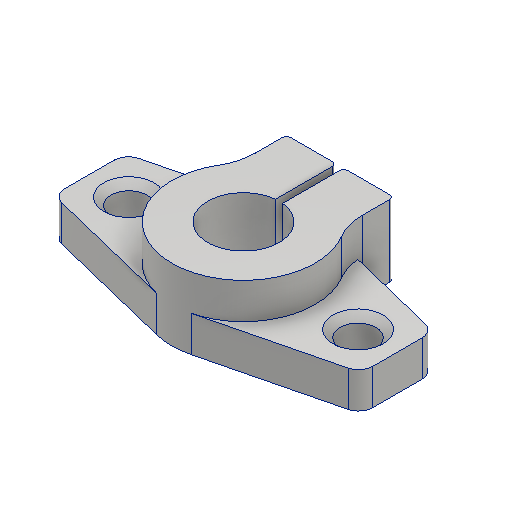
# Autodesk Inventor part: COTS_GENERIC_SHF10_Linear_Rail_Mount
Saved by Autodesk Inventor 2026.1 (Build 301233000, 233)
## iProperties
Created: 2017-05-24
Part Number: COTS_GENERIC_SHF10_Linear_Rail_Mount
Material: Ogólny
Document SubType Name: Modeling
Designer: Andrzej
Density: 1 g/cm^3
Appearance: Aluminium - płaski
Author: Andrzej
Autodesk Inventor part; units mm, degrees
ref_plane "YZ Plane" through (0, 0, 0) normal (1, 0, 0) x (0, 1, 0)
ref_plane "XZ Plane" through (0, 0, 0) normal (0, 1, 0) x (-1, 0, 0)
ref_plane "XY Plane" through (0, 0, 0) normal (0, 0, 1) x (1, 0, 0)
sketch "Szkic1" plane through (0, 0, 0) normal (0, 0, 1) x (1, 0, 0)
  circle A0 centre (0, 0) radius 5
  line L0 (-21.5, 5) -> (-21.5, -5)
  line L1 (21.5, 5) -> (21.5, -5)
  circle A1 centre (0, 0) radius 10
  line L2 (-21.5, -5) -> (-2.3932, -9.7094)
  line L3 (21.5, -5) -> (2.3932, -9.7094)
  line L4 (-7.5, 13.5) -> (7.5, 13.5)
  line L5 (-21.5, 5) -> (-7.5, 8.4507)
  line L6 (21.5, 5) -> (7.5, 8.4507)
  line L7 (-7.5, 13.5) -> (-7.5, 6.6144)
  line L8 (7.5, 13.5) -> (7.5, 6.6144)
  dimension "d0" = 10
  dimension "d1" = 43
  dimension "d2" = 10
  dimension "d3" = 10
  dimension "d4" = 5
  dimension "d5" = 21.5
  dimension "d6" = 20
  dimension "d7" = 13.5
  dimension "d8" = 7.5
  dimension "d9" = 15
  constraints: 18 end point, 4 point on circle, 4 tangent, 3 vertical, 2 centre point, 2 coincident, 2 point on line, 1 horizontal, 1 parallel
  measures "d0" diameter of A0
  measures "d1" distance between parallel lines of L1 L0
  measures "d2" distance of L0.start L0.end
  measures "d3" distance of L1.start L1.end
  measures "d4" vertical distance of point (0, 0) L0.start
  measures "d5" distance from line of point (0, 0) L0
  measures "d6" diameter of A1
  measures "d7" distance from line of point (0, 0) L4
  measures "d8" horizontal distance of point (0, 0) L4.start
  measures "d9" distance of L4.start L4.end
extrude "Wyciągnięcie proste1" add sketch "Szkic1" along normal blind 5 contours L5 L7 A1 L2 L0 | A1 L8 L6 L1 L3
extrude "Wyciągnięcie proste2" add sketch "Szkic1" along normal blind 10 contours L7 L4 L8 A1 | A1
fillet "Zaokrąglenie1" radius 8 2 edges at (7.5, 6.6144, 7.5) (-7.5, 6.6144, 7.5)
fillet "Zaokrąglenie2" radius 2 4 edges at (21.5, 5, 2.5) (21.5, -5, 2.5) (-21.5, -5, 2.5) (-21.5, 5, 2.5)
sketch "Szkic2" plane through (0, 0, 10) normal (0, 0, 1) x (1, 0, 0)
  line L0 (-0.5, 2.515) -> (0.5, 2.515)
  line L1 (0.5, 2.515) -> (0.5, 16.0792)
  line L2 (0.5, 16.0792) -> (-0.5, 16.0792)
  line L3 (-0.5, 16.0792) -> (-0.5, 2.515)
  point P0 (0, 0)
  dimension "d16" = 1
  dimension "d17" = 0.5
  constraints: 8 end point, 2 parallel, 1 horizontal, 1 perpendicular
  measures "d16" distance of L2.end L1.end
  measures "d17" distance from line of point (0, 0) L3
extrude "Wyciągnięcie proste3" cut sketch "Szkic2" against normal through all
fillet "Zaokrąglenie3" radius 0.6 4 edges at (-7.5, 13.5, 5) (-0.5, 13.5, 5) (0.5, 13.5, 5) (7.5, 13.5, 5)
sketch "Szkic3" plane through (0, 0, 5) normal (0, 0, 1) x (1, 0, 0)
  arc A0 (-19.9786, 5.375) -> (-21.5, 3.4331) centre (-19.5, 3.4331) ccw projected
  line L0 (-21.5, 3.4331) -> (-21.5, -3.4331) projected
  arc A1 (-21.5, -3.4331) -> (-19.9786, -5.375) centre (-19.5, -3.4331) ccw projected
  line L1 (-19.9786, -5.375) -> (-2.3932, -9.7094) projected
  arc A2 (-8.6111, 5.0842) -> (-2.3932, -9.7094) centre (0, 0) ccw projected
  arc A3 (-8.6111, 5.0842) -> (-7.5314, 8.4429) centre (-15.5, 9.1515) ccw projected
  line L2 (-7.5314, 8.4429) -> (-19.9786, 5.375) projected
  arc A4 (19.9786, -5.375) -> (21.5, -3.4331) centre (19.5, -3.4331) ccw projected
  line L3 (21.5, -3.4331) -> (21.5, 3.4331) projected
  arc A5 (21.5, 3.4331) -> (19.9786, 5.375) centre (19.5, 3.4331) ccw projected
  line L4 (19.9786, 5.375) -> (7.5314, 8.4429) projected
  arc A6 (7.5314, 8.4429) -> (8.6111, 5.0842) centre (15.5, 9.1515) ccw projected
  arc A7 (2.3932, -9.7094) -> (8.6111, 5.0842) centre (0, 0) ccw projected
  line L5 (2.3932, -9.7094) -> (19.9786, -5.375) projected
  point P0 (-16, 0)
  point P1 (16, 0)
  dimension "d21" = 32
  dimension "d22" = 43
  dimension "d23" = 5.5
  measures "d21" distance of point (16, 0) point (-16, 0)
  measures "d22" distance between parallel lines of L3 L0
  measures "d23" distance from line of L0 point (-16, 0)
hole "Otwór1" at (-16, 0, 5) at (16, 0, 5) direction (0, 0, -1) diameter 5 end through all
chamfer "Faza1" distance 1 angle 45 2 edges at (-16, 2.5, 5) (16, 2.5, 5)
equation "\"d3\" = d2"
equation "\"d5\" = 0.5 * d1"
equation "\"d8\" = 0.5 * d9"
equation "\"d23\" = -0.5 * d21 + 0.5 * d22"
